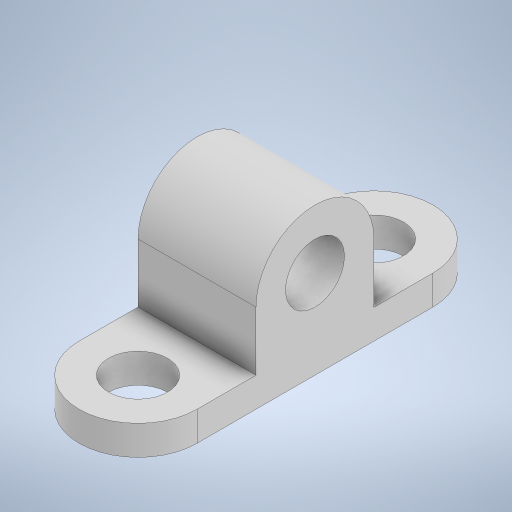
# Autodesk Inventor part: tarea de practica dinamica
Saved by Autodesk Inventor 2023 (Build 270158000, 158)
## iProperties
Created: 2024-01-30
Part Number: tarea de practica dinamica
Material: Generic
Document SubType Name: Modeling
Designer: Usuario
Density: 1 g/cm^3
Appearance: Default
Author: Usuario
Autodesk Inventor part; units mm, degrees
ref_plane "YZ Plane" through (0, 0, 0) normal (1, 0, 0) x (0, 1, 0)
ref_plane "XZ Plane" through (0, 0, 0) normal (0, 1, 0) x (-1, 0, 0)
ref_plane "XY Plane" through (0, 0, 0) normal (0, 0, 1) x (1, 0, 0)
sketch "Sketch1" plane through (0, 0, 0) normal (0, 1, 0) x (-1, 0, 0)
  line L0 (-20, 20) -> (-20, -20)
  line L1 (20, -20) -> (20, 20)
  circle A0 centre (0, 40) radius 10
  circle A1 centre (0, -40) radius 10
  arc A2 (20, 40) -> (-20, 40) centre (0, 40) ccw
  arc A3 (-20, -40) -> (20, -40) centre (0, -40) ccw
  line L2 (20, 40) -> (20, 20)
  line L3 (20, -20) -> (20, -40)
  line L4 (-20, -40) -> (-20, -20)
  line L5 (-20, 20) -> (-20, 40)
  point P0 (0, 0)
  constraints: 12 end point, 4 centre point, 4 point on circle, 2 parallel, 2 point on line, 1 coincident, 1 tangent, 1 vertical
extrude "Extrusion1" add sketch "Sketch1" along normal blind 10
sketch "Sketch2" plane through (20, 0, 40) normal (1, 0, 0) x (0, 0, -1)
  circle A0 centre (40, 30) radius 10
  arc A1 (60, 30) -> (20, 30) centre (40, 30) ccw
  line L0 (20, 30) -> (20, 10)
  line L1 (0, 10) -> (80, 10) projected
  line L2 (60, 30) -> (60, 10)
  point P0 (40, 0)
  constraints: 4 end point, 2 centre point, 2 point on circle, 2 point on line, 1 coincident, 1 parallel, 1 vertical
extrude "Extrusion2" add sketch "Sketch2" against normal blind 40
body "Solid1"
